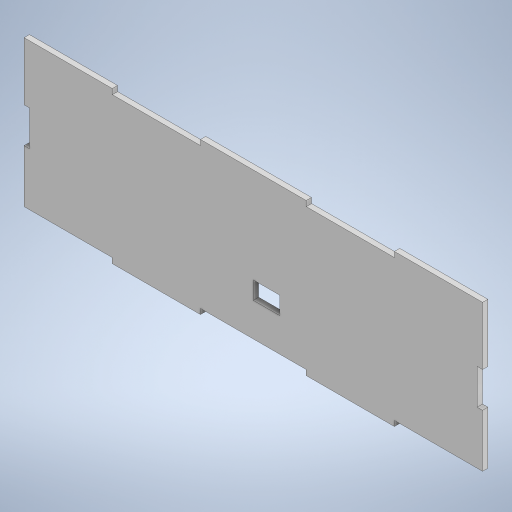
# Autodesk Inventor part: Belakang
Saved by Autodesk Inventor 2024 (Build 280153000, 153)
## iProperties
Created: 2023-08-09
Part Number: Belakang
Material: Generic
Document SubType Name: Modeling
Designer: Asus
Density: 1 g/cm^3
Appearance: Default
Author: Asus
Autodesk Inventor part; units mm, degrees
ref_plane "YZ Plane" through (0, 0, 0) normal (1, 0, 0) x (0, 1, 0)
ref_plane "XZ Plane" through (0, 0, 0) normal (0, 1, 0) x (-1, 0, 0)
ref_plane "XY Plane" through (0, 0, 0) normal (0, 0, 1) x (1, 0, 0)
sketch "Sketch1" plane through (0, 0, 0) normal (0, 0, 1) x (1, 0, 0)
  line L0 (0, 0) -> (0, 3) construction
  line L1 (0, 3) -> (50, 3)
  line L2 (50, 3) -> (50, 0)
  line L3 (50, 0) -> (100, 0)
  line L4 (100, 0) -> (100, 3)
  line L5 (100, 3) -> (160, 3)
  line L6 (160, 3) -> (160, 0)
  line L7 (160, 0) -> (210, 0)
  line L8 (210, 0) -> (210, 3)
  line L9 (210, 3) -> (260, 3)
  line L10 (260, 3) -> (260, 33)
  line L11 (260, 33) -> (257, 33)
  line L12 (257, 33) -> (257, 53)
  line L13 (257, 53) -> (260, 53)
  line L14 (260, 53) -> (260, 86)
  line L15 (0, 86) -> (0, 53)
  line L16 (0, 53) -> (3, 53)
  line L17 (3, 53) -> (3, 33)
  line L18 (3, 33) -> (0, 33)
  line L19 (0, 33) -> (0, 3)
  line L20 (260, 0) -> (260, 25) construction
  line L21 (260, 25) -> (260, 28) construction
  line L22 (135, 28) -> (135, 0) construction
  line L23 (135, 0) -> (135, 20) construction
  line L24 (130, 28) -> (130, 0) construction
  line L25 (130, 0) -> (130, 25) construction
  line L26 (260, 0) -> (260, 22) construction
  line L27 (260, 22) -> (260, 32) construction
  line L28 (260, 32) -> (145, 32) construction
  line L29 (145, 32) -> (130, 32) construction
  line L30 (130, 32) -> (130, 22)
  line L31 (145, 22) -> (145, 32)
  line L32 (130, 32) -> (145, 32)
  line L33 (130, 22) -> (145, 22)
  line L34 (260, 86) -> (210, 86)
  line L35 (210, 86) -> (210, 83)
  line L36 (210, 83) -> (160, 83)
  line L37 (160, 83) -> (160, 86)
  line L38 (160, 86) -> (100, 86)
  line L39 (100, 86) -> (100, 83)
  line L40 (100, 83) -> (50, 83)
  line L41 (50, 83) -> (50, 86)
  line L42 (50, 86) -> (0, 86)
  point P0 (0, 18)
  dimension "d0" = 3
  dimension "d2" = 50
  dimension "d3" = 60
  dimension "d4" = 50
  dimension "d5" = 50
  dimension "d6" = 30
  dimension "d7" = 3
  dimension "d8" = 20
  dimension "d9" = 33
  dimension "d10" = 33
  dimension "d11" = 3
  dimension "d12" = 20
  dimension "d24" = 20
  dimension "d29" = 25
  dimension "d32" = 22
  dimension "d33" = 10
  dimension "d34" = 115
  dimension "d35" = 15
  dimension "d37" = 3
  dimension "d38" = 50
  dimension "d39" = 3
  dimension "d40" = 50
  dimension "d41" = 50
  constraints: 86 end point, 26 point on line, 16 perpendicular, 3 equal length, 2 horizontal, 2 vertical, 1 midpoint
  measures "d0" distance of L0.start L0.end
  measures "d2" distance of L2.end L3.end
  measures "d3" distance of L4.end L5.end
  measures "d4" distance of L6.end L7.end
  measures "d5" distance of L8.end L9.end
  measures "d6" distance of L9.end L10.end
  measures "d7" distance of L10.end L11.end
  measures "d8" distance of L11.end L12.end
  measures "d9" distance of L13.end L14.end
  measures "d10" distance of L15.start L15.end
  measures "d11" distance of L15.end L16.end
  measures "d12" distance of L16.end L17.end
  measures "d24" distance of L22.end L23.end
  measures "d29" distance of L24.end L25.end
  measures "d32" distance of L20.start L26.end
  measures "d33" distance of L26.end L27.end
  measures "d34" distance of L27.end L28.end
  measures "d35" distance of L28.end L29.end
  measures "d37" distance of L34.end L35.end
  measures "d38" distance of L35.end L36.end
  measures "d39" distance of L36.end L37.end
  measures "d40" distance of L39.end L40.end
  measures "d41" distance of L0.end L1.end
extrude "Extrusion1" add sketch "Sketch1" along normal blind 3
body "Solid1"
